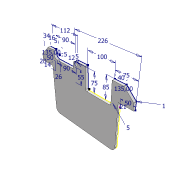
# Autodesk Inventor part: SlipersLåda 211018003
Saved by Autodesk Inventor 2020 (Build 240168000, 168)
## iProperties
Created: 2021-10-18
Part Number: SlipersLåda 211018003
Material: Generic
Document SubType Name: Modeling
Designer: dicpet001
Density: 1 g/cm^3
Appearance: Default
Author: dicpet001
Autodesk Inventor part; units mm, degrees
ref_plane "YZ Plane" through (0, 0, 0) normal (1, 0, 0) x (0, 1, 0)
ref_plane "XZ Plane" through (0, 0, 0) normal (0, 1, 0) x (-1, 0, 0)
ref_plane "XY Plane" through (0, 0, 0) normal (0, 0, 1) x (1, 0, 0)
sketch "Sketch1" plane through (0, 0, 0) normal (0, 0, 1) x (1, 0, 0)
  line L0 (0, 118.387) -> (0, -122.322) projected
  line L1 (-200.109, 0) -> (200.109, 0) projected
  line L2 (-139, 84) -> (139, 84)
  line L3 (139, 84) -> (139, -65)
  line L4 (120, -84) -> (-120, -84)
  line L5 (-139, -65) -> (-139, 84)
  arc A0 (-139, -65) -> (-120, -84) centre (-120, -65) ccw
  arc A1 (120, -84) -> (139, -65) centre (120, -65) ccw
  point P0 (0, 0)
  dimension "d0" = 278
  dimension "d1" = 168
  dimension "d2" = 19
  constraints: 8 end point, 4 point on circle, 4 tangent, 2 centre point, 2 parallel, 1 equal radius, 1 horizontal, 1 perpendicular, 2 other
  measures "d0" distance between parallel lines of L3 L5
  measures "d1" distance between parallel lines of L2 L4
  measures "d2" radius of A0
extrude "Extrusion1" add sketch "Sketch1" against normal blind 10
sketch "Sketch2" plane through (0, 0, -10) normal (0, 0, -1) x (-1, 0, 0)
  line L0 (139, -65) -> (139, 84) projected
  line L1 (139, 84) -> (-139, 84) projected
  line L2 (-139, 84) -> (-139, -65) projected
  arc A0 (-139, -65) -> (-120, -84) centre (-120, -65) ccw projected
  line L3 (-120, -84) -> (120, -84) projected
  arc A1 (120, -84) -> (139, -65) centre (120, -65) ccw projected
  line L4 (-139, 84) -> (-139, 105)
  line L5 (-139, 105) -> (-188, 105)
  line L6 (-189, 106) -> (-189, 133.5858)
  line L7 (-188.7071, 134.2929) -> (-154.2929, 168.7071)
  line L8 (-153.5858, 169) -> (-115, 169)
  line L9 (-114, 168) -> (-114, 89)
  line L10 (-14, 89) -> (-14, 168)
  line L11 (-13, 169) -> (27, 169)
  line L12 (37, 159) -> (37, 144)
  line L13 (42, 139) -> (113, 139)
  line L14 (139, 84) -> (139, 104)
  line L15 (189, 104) -> (189, 135)
  line L16 (189, 135) -> (155, 169)
  line L17 (155, 169) -> (132, 169)
  arc A2 (-114, 89) -> (-109, 84) centre (-109, 89) ccw
  arc A3 (-19, 84) -> (-14, 89) centre (-19, 89) ccw
  arc A4 (-188.7071, 134.2929) -> (-189, 133.5858) centre (-188, 133.5858) ccw
  arc A5 (-189, 106) -> (-188, 105) centre (-188, 106) ccw
  arc A6 (-153.5858, 169) -> (-154.2929, 168.7071) centre (-153.5858, 168) ccw
  arc A7 (-114, 168) -> (-115, 169) centre (-115, 168) ccw
  arc A8 (-13, 169) -> (-14, 168) centre (-13, 168) ccw
  arc A9 (113, 139) -> (127, 153) centre (113, 153) ccw
  arc A10 (37, 144) -> (42, 139) centre (42, 144) ccw
  line L18 (127, 164) -> (127, 153)
  line L19 (139, 104) -> (189, 104)
  circle A11 centre (27, 159) radius 6
  arc A12 (37, 159) -> (27, 169) centre (27, 159) ccw
  line L20 (132, 169) -> (127, 164)
  line L21 (-139, 84) -> (-135, 84) projected
  line L22 (-139, 84) -> (-109, 84)
  line L23 (-139, 84) -> (139, 84) projected
  line L24 (-19, 84) -> (139, 84)
  point P0 (0, 0)
  point P1 (-189, 105)
  point P2 (-154, 169)
  point P3 (-14, 169)
  point P4 (37, 139)
  point P5 (127, 139)
  point P6 (127, 169)
  point P7 (135, 84)
  dimension "d8" = 21
  dimension "d9" = 50
  dimension "d10" = 85
  dimension "d11" = 75
  dimension "d12" = 135
  dimension "d13" = 40
  dimension "d14" = 100
  dimension "d16" = 90
  dimension "d17" = 50
  dimension "d19" = 34
  dimension "d20" = 135
  dimension "d21" = 5
  dimension "d22" = 1
  dimension "d23" = 14
  dimension "d24" = 5
  dimension "d26" = 90
  dimension "d29" = 12
  dimension "d30" = 226
  dimension "d31" = 5
  dimension "d32" = 5
  dimension "d33" = 55
  dimension "d34" = 20
  dimension "d35" = 16
  dimension "d36" = 75
  dimension "d37" = 112
  dimension "d38" = 26
  constraints: 38 end point, 20 point on circle, 16 tangent, 12 point on line, 11 centre point, 5 equal radius, 4 perpendicular, 4 vertical, 3 collinear, 2 horizontal, 1 coincident, 1 parallel
  measures "d8" distance of L1.end L4.end
  measures "d9" distance of L4.end point (-189, 105)
  measures "d10" distance between parallel lines of L1 L8
  measures "d11" distance between parallel lines of L9 L6
  measures "d12" angle of L8 L7
  measures "d13" distance from line of L9 point (-154, 169)
  measures "d14" distance between parallel lines of L10 L9
  measures "d16" distance of point (37, 139) point (127, 139)
  measures "d17" distance of L14.end L15.start
  measures "d19" distance from line of L15 L16.end
  measures "d20" angle of L16 L17
  measures "d21" radius of A2
  measures "d22" radius of A4
  measures "d23" radius of A9
  measures "d24" radius of A10
  measures "d26" distance between parallel lines of L18 L12
  measures "d29" diameter of A11
  measures "d30" distance between parallel lines of L12 L6
  measures "d31" distance of L17.end point (127, 169)
  measures "d32" distance of L18.start point (127, 169)
  measures "d33" distance between parallel lines of L13 L1
  measures "d34" distance between parallel lines of L1 L19
  measures "d35" distance from line of L16.end L0
  measures "d36" distance from line of L1 A11.centre
  measures "d37" distance from line of A11.centre L0
  measures "d38" distance from line of A9.centre L0
extrude "Extrusion2" add sketch "Sketch2" against normal blind 10 contours L1 A3 L10 A8 L11 A12 L12 A10 L13 A9 L18 L20 L17 L16 L15 L19 L14 | L1 L4 L5 A5 L6 A4 L7 A6 L8 A7 L9 A2
chamfer "Chamfer2" distance 4 angle 45 6 edges at (139, 20, -10) (133.435, -78.435, -10) (0, -84, -10) (-133.435, -78.435, -10) (-139, 19.5, -10) (-164, 104, -10)
chamfer "Chamfer3" distance 4 angle 45 1 edges at (-164, 104, 0)
sketch "Sketch3" plane through (189, 106, -10) normal (1, 0, 0) x (0, 0, -1)
  line L0 (0, 27.5858) -> (0, 0) projected
  line L1 (0, 27.5858) -> (-10, 27.5858) projected
  line L2 (-10, 0) -> (-10, 27.5858) projected
  line L3 (0, 0) -> (-10, 0) projected
  line L4 (0, 0) -> (0, -1) projected
  line L5 (0, 0) -> (-10, 0) projected
  line L6 (-10, -1) -> (-10, 0) projected
  line L7 (0, -1) -> (-10, -1) projected
  line L8 (-10, 3) -> (-6, -1)
  line L9 (-10, 3) -> (-10, -1)
  line L10 (0, -1) -> (-10, -1) projected
  line L11 (-10, -1) -> (-6, -1)
  line L12 (-5, -1) -> (-5, 5.9932)
  line L13 (0, -1) -> (0, 0)
  line L14 (0, 3) -> (-4, -1)
  line L15 (0, 3) -> (0, -1)
  line L16 (0, -1) -> (-4, -1)
  point P0 (-10, -106)
  point P1 (-10, 3)
  point P2 (0, 3)
  dimension "d47" = 45
  dimension "d48" = 4
  constraints: 16 end point, 4 symmetric about line, 3 point on line, 2 collinear, 1 midpoint, 1 vertical
  measures "d47" angle of L8 L7
  measures "d48" distance from line of L8.end L6
extrude "Extrusion3" cut sketch "Sketch3" against normal up to surface (50 mm away) contours L0 L3 L14 | L4 L7 L14 L3 | L8 L3 L2 | L3 L8 L7 L6
ref_plane "Work Plane1" through (139, 109, -10) normal (-0.5773503, 0.5773503, 0.5773503) x (-0.7071068, -0.7071068, 0)
sketch "Sketch4" plane through (139, 109, -10) normal (-0.5773503, 0.5773503, 0.5773503) x (-0.7071068, -0.7071068, 0)
  line L0 (2.8284, 4.899) -> (-31.8198, 24.9031) projected
  line L1 (5.6569, 0) -> (2.8284, 4.899) projected
  line L2 (-35.3553, 20.4124) -> (0, 0) projected
  line L3 (2.8284, 4.899) -> (0, 0)
  line L4 (0, 0) -> (5.6569, 0)
  line L5 (5.6569, 0) -> (2.8284, 4.899)
  point P0 (175.3625, -4.0825)
  constraints: 6 end point, 1 horizontal, 1 perpendicular
extrude "Extrusion4" cut sketch "Sketch4" against normal blind 10
move faces "Move1" translate (0, 1, 0) faces at (-172.3333, 104, -4.6667) (-155.6667, 105.3333, -2.6667) (-154.3333, 106.6667, -8.6667)
equation "\"d32\" = d31"
body "Solid1"
